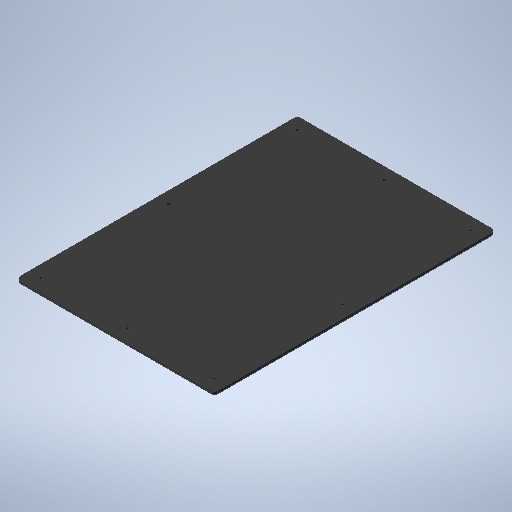
# Autodesk Inventor part: BED_PLATE_V2
Saved by Autodesk Inventor 2025.2 (Build 292293000, 293)
## iProperties
Created: 2026-03-27
Part Number: BED_PLATE_V2
Material: Generic
Document SubType Name: Modeling
Designer: composite
Density: 1 g/cm^3
Appearance: Default
Author: composite
Autodesk Inventor part; units mm, degrees
ref_plane "YZ Plane" through (0, 0, 0) normal (1, 0, 0) x (0, 1, 0)
ref_plane "XZ Plane" through (0, 0, 0) normal (0, 1, 0) x (-1, 0, 0)
ref_plane "XY Plane" through (0, 0, 0) normal (0, 0, 1) x (1, 0, 0)
sketch "Sketch1" plane through (0, 0, 0) normal (0, 1, 0) x (-1, 0, 0)
  line L0 (0, 0) -> (335.5, 0)
  line L1 (335.5, 0) -> (335.5, -476)
  line L2 (335.5, -476) -> (0, -476)
  line L3 (0, -476) -> (0, 0)
  circle A0 centre (315.5, -20) radius 3
  circle A1 centre (315.5, -456) radius 3
  circle A2 centre (20, -20) radius 3
  circle A3 centre (20, -456) radius 3
  circle A4 centre (167.75, -20) radius 3
  circle A5 centre (167.75, -456) radius 3
  circle A6 centre (315.5, -238) radius 3
  circle A7 centre (20, -238) radius 3
  point P0 (167.75, 0)
  point P1 (167.75, -476)
  point P2 (0, -238)
  point P3 (335.5, -238)
  dimension "d0" = 335.5
  dimension "d1" = 476
  dimension "d2" = 6
  dimension "d3" = 20
  dimension "d4" = 20
  dimension "d7" = 436
  dimension "d10" = 295.5
  dimension "d13" = 6
  dimension "d14" = 6
  dimension "d15" = 6
  dimension "d16" = 6
  constraints: 8 centre point, 8 end point, 4 horizontal alignment, 4 midpoint, 4 vertical alignment, 2 horizontal, 2 parallel, 1 perpendicular, 1 vertical, 6 other
  measures "d0" distance of L1.end L2.end
  measures "d1" distance of L0.end L1.end
  measures "d2" diameter of A0
  measures "d3" distance from line of L1 A0.centre
  measures "d4" distance from line of A0.centre L0
  measures "d7" distance of A0.centre A1.centre
  measures "d10" distance of A0.centre A2.centre
  measures "d13" diameter of A5
  measures "d14" diameter of A4
  measures "d15" diameter of A6
  measures "d16" diameter of A7
extrude "Extrusion1" add sketch "Sketch1" along normal blind 5
fillet "Fillet1" radius 5 4 edges at (0, 2.5, 0) (-335.5, 2.5, 0) (-335.5, 2.5, -476) (0, 2.5, -476)
equation "\"d14\" = d2"
body "Solid1"
